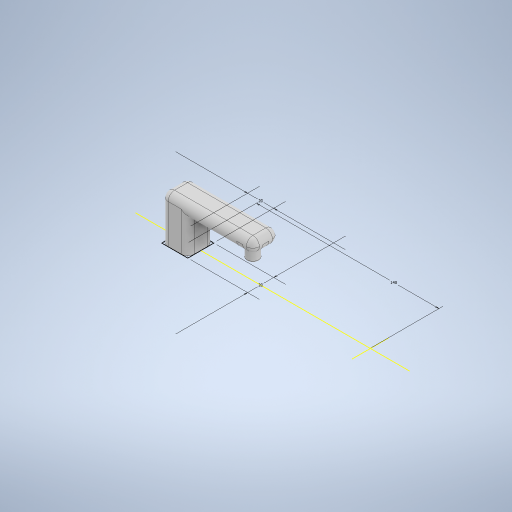
# Autodesk Inventor part: uMule-uchwyt_servo
Saved by Autodesk Inventor 2024.2 (Build 282272000, 272)
## iProperties
Created: 2024-10-20
Part Number: uMule-uchwyt_servo
Material: Ogólny
Document SubType Name: Modeling
Designer: owozn
Density: 1 g/cm^3
Appearance: Domyślna
Author: owozn
Autodesk Inventor part; units mm, degrees
ref_plane "YZ Plane" through (0, 0, 0) normal (1, 0, 0) x (0, 1, 0)
ref_plane "XZ Plane" through (0, 0, 0) normal (0, 1, 0) x (-1, 0, 0)
ref_plane "XY Plane" through (0, 0, 0) normal (0, 0, 1) x (1, 0, 0)
sketch "Szkic1" plane through (0, 0, 0) normal (0, 1, 0) x (-1, 0, 0)
  line L0 (180, 0) -> (-30, 0) projected
  line L1 (0, -14) -> (0, 14) projected
  line L2 (150, 10) -> (130, 10)
  line L3 (130, 10) -> (130, -10)
  line L4 (130, -10) -> (150, -10)
  line L5 (150, -10) -> (150, 10)
  line L6 (150, 10) -> (130, -10) construction
  line L7 (130, 10) -> (150, -10) construction
  point P0 (0, 0)
  point P1 (140, 0)
  dimension "d3" = 20
  dimension "d4" = 20
  dimension "d5" = 140
  constraints: 12 end point, 2 midpoint, 2 parallel, 1 horizontal, 1 perpendicular, 1 point on line
  measures "d3" distance of L4.end L3.end
  measures "d4" distance of L3.end L2.end
  measures "d5" distance of point (0, 0) point (140, 0)
extrude "Wyciągnięcie proste1" add sketch "Szkic1" along normal blind 35
sketch "Szkic2" plane through (-130, 0, 10) normal (1, 0, 0) x (0, 0, -1)
  line L0 (10, -7) -> (10, 42) projected
  line L1 (24, 0) -> (-4, 0) projected
  line L2 (0, 35) -> (20, 35)
  line L3 (20, 35) -> (20, 25)
  line L4 (20, 25) -> (0, 25)
  line L5 (0, 25) -> (0, 35)
  line L6 (0, 35) -> (20, 25) construction
  line L7 (20, 35) -> (0, 25) construction
  line L8 (0, 0) -> (20, 0) projected
  point P0 (10, 0)
  point P1 (10, 30)
  point P2 (10, 0)
  dimension "d8" = 20
  dimension "d9" = 10
  dimension "d10" = 30
  constraints: 12 end point, 3 midpoint, 2 parallel, 1 horizontal, 1 perpendicular, 1 point on line
  measures "d8" distance of L3.end L4.end
  measures "d9" distance of L2.end L3.end
  measures "d10" distance of point (10, 0) point (10, 30)
extrude "Wyciągnięcie proste2" add sketch "Szkic2" along normal blind 50
sketch "Szkic3" plane through (-130, 25, -10) normal (0, -1, 0) x (1, 0, 0)
  circle A0 centre (40, 10) radius 4.5
  line L0 (130, -4) -> (130, 24) projected
  line L1 (-50, 10) -> (160, 10) projected
  point P0 (130, 10)
  dimension "d13" = 9
  dimension "d14" = 90
  constraints: 1 centre point, 1 point on line
  measures "d13" diameter of A0
  measures "d14" distance of point (130, 10) A0.centre
extrude "Wyciągnięcie proste3" add sketch "Szkic3" along normal blind 10
fillet "Zaokrąglenie1" radius 1 2 edges at (-94.5, 15, 0) (-94.5, 25, 0)
fillet "Zaokrąglenie2" radius 5 13 edges at (-105, 25, 10) (-130, 12.5, 10) (-130, 12.5, -10) (-105, 25, -10) (-115, 35, 10) (-150, 17.5, -10) (-150, 17.5, 10) (-115, 35, -10) (-80, 25, 0) (-80, 35, 0) (-80, 30, -10) (-80, 30, 10) (-150, 35, 0)
